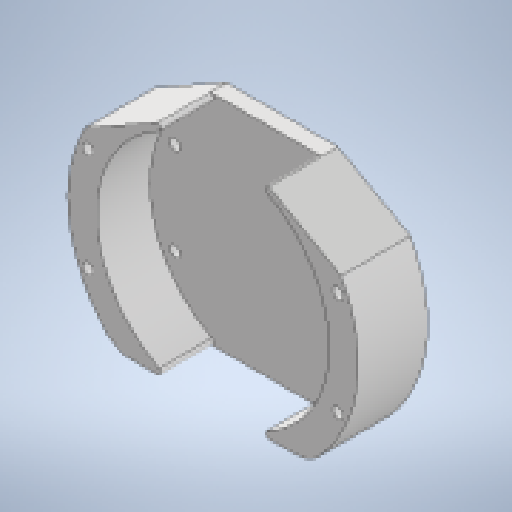
# Autodesk Inventor part: basefixpart_forR6
Saved by Autodesk Inventor 2024.3 (Build 283343010, 343A)
## iProperties
Created: 2025-05-24
Part Number: basefixpart_forR6
Material: 一般
Document SubType Name: Modeling
Designer: kshau
Density: 1 g/cm^3
Appearance: 既定
Mass: 77.9972 g
Surface Area: 271.132 cm^2
Volume: 77.9972 cm^3
Author: kshau
Autodesk Inventor part; units mm, degrees
ref_plane "YZ Plane" through (0, 0, 0) normal (1, 0, 0) x (0, 1, 0)
ref_plane "XZ Plane" through (0, 0, 0) normal (0, 1, 0) x (-1, 0, 0)
ref_plane "XY Plane" through (0, 0, 0) normal (0, 0, 1) x (1, 0, 0)
sketch "スケッチ1" plane through (0, 0, 0) normal (0, 0, 1) x (1, 0, 0)
  circle A0 centre (0, 0) radius 44
  line L0 (0, 0) -> (44, 0)
  line L1 (0, 0) -> (28.9895, 33.1)
  line L2 (28.9895, 33.1) -> (0, 33.1)
  line L3 (0, 0) -> (0, 44)
  line L4 (-28.9895, 33.1) -> (0, 33.1)
  line L5 (28.9895, -33.1) -> (0, -33.1)
  line L6 (-28.9895, -33.1) -> (0, -33.1)
  line L7 (15.4, -33.1) -> (15.4, -41.217)
  line L8 (-15.4, -33.1) -> (-15.4, -41.217)
  line L9 (15.4, 33.1) -> (15.4, 41.217)
  line L10 (-15.4, 33.1) -> (-15.4, 41.217)
  point P0 (-28.9895, 33.1)
  point P1 (-28.9895, -33.1)
  point P2 (28.9895, -33.1)
  point P3 (15.4, 33.1)
  point P4 (-15.4, 33.1)
  point P5 (-15.4, -33.1)
  dimension "d0" = 88
  dimension "d20" = 15.4
  dimension "d21" = 33.1
  constraints: 22 end point, 10 symmetric about line, 4 point on circle, 2 horizontal, 1 centre point, 1 coincident, 1 perpendicular, 1 point on line, 1 vertical
  measures "d0" diameter of A0
  measures "d20" distance between parallel lines of L3 L7
  measures "d21" distance between parallel lines of L0 L2
extrude "押し出し1" add sketch "スケッチ1" along normal blind 5
sketch "スケッチ13" plane through (0, 0, 5) normal (0, 0, 1) x (1, 0, 0)
  circle A0 centre (0, 0) radius 44
  circle A1 centre (0, 0) radius 35.25
  circle A2 centre (0, 0) radius 44 projected
  line L0 (0, 44) -> (0, 0)
  line L1 (7.85, 43.2941) -> (7.85, -43.2941)
  line L2 (-7.85, 43.2941) -> (-7.85, -43.2941)
  point P0 (7.85, -34.3648)
  point P1 (7.85, -43.2941)
  point P2 (7.85, 34.3648)
  point P3 (-7.85, -34.3648)
  point P4 (-7.85, 34.3648)
  dimension "d76" = 88
  dimension "d77" = 70.5
  dimension "d78" = 7.85
  constraints: 6 end point, 3 point on circle, 2 centre point, 2 coincident, 2 symmetric about line, 2 vertical
  measures "d76" diameter of A0
  measures "d77" diameter of A1
  measures "d78" distance between parallel lines of L0 L1
extrude "押し出し9" add sketch "スケッチ13" along normal blind 16 contours A0 L1 A1 | L1 A1 L0 A0 | A0 L2 A1 L1 | L0 A1 L2 A0 | A0 L2 A1
sketch "スケッチ16" plane through (0, 0, 0) normal (0, 0, -1) x (-1, 0, 0)
  line L0 (0, 0) -> (-44, 0)
  circle A0 centre (0, 0) radius 44 projected
  line L1 (0, 0) -> (-40.6507, 16.8381)
  circle A1 centre (0, 0) radius 41
  point P0 (-7.85, -43.2941)
  point P1 (-7.85, 43.2941)
  point P2 (-37.8791, 15.69)
  point P3 (-37.8791, -15.69)
  point P4 (-15.69, -37.8791)
  point P5 (15.69, -37.8791)
  point P6 (37.8791, -15.69)
  point P7 (37.8791, 15.69)
  point P8 (15.69, 37.8791)
  point P9 (-15.69, 37.8791)
  dimension "d92" = 82
  dimension "d91" = 22.5
  dimension "d95" = 360
  constraints: 4 end point, 2 point on circle, 1 coincident, 1 horizontal, 1 point on line, 12 other
  measures "d91" angle of L0 L1
hole "穴5" at (37.8791, 15.69, 0) at (37.8791, -15.69, 0) at (-37.8791, -15.69, 0) at (-37.8791, 15.69, 0) direction (0, 0, 1) diameter 3.3 end through all
sketch "スケッチ19" plane through (0, 0, 0) normal (0, 0, -1) x (-1, 0, 0)
  circle A0 centre (0, 0) radius 31
  line L0 (0, 0) -> (44, 0)
  circle A1 centre (0, 0) radius 44 projected
  line L1 (0, 0) -> (0, 31)
  point P0 (27.6333, 14.05)
  point P1 (27.6333, -14.05)
  point P2 (-27.6333, 14.05)
  point P3 (-27.6333, -14.05)
  dimension "d129" = 62
  dimension "d130" = 14.05
  constraints: 4 end point, 3 symmetric about line, 2 point on circle, 1 centre point, 1 coincident, 1 horizontal, 1 horizontal alignment, 1 vertical, 1 other
  measures "d129" diameter of A0
  measures "d130" distance from line of L0 A0.start
hole "穴6" at (-27.6333, 14.05, 0) at (-27.6333, -14.05, 0) at (27.6333, -14.05, 0) at (27.6333, 14.05, 0) direction (0, 0, 1) diameter 3.3 end through all
sketch "スケッチ21" plane through (0, 0, 0) normal (0, 0, -1) x (-1, 0, 0)
  circle A0 centre (0, 0) radius 17.5
  dimension "d143" = 35
  constraints: 1 centre point, 1 coincident
  measures "d143" diameter of A0
extrude "押し出し15" add sketch "スケッチ21" along normal blind 5
sketch "スケッチ22" plane through (0, 0, -5) normal (0, 0, -1) x (-1, 0, 0)
  circle A0 centre (0, 0) radius 11.15
  dimension "d146" = 22.3
  constraints: 1 centre point, 1 coincident
  measures "d146" diameter of A0
extrude "押し出し16" cut sketch "スケッチ22" against normal blind 6
sketch "スケッチ23" plane through (0, 0, 21) normal (0, 0, 1) x (1, 0, 0)
  circle A0 centre (0, 0) radius 11.15 projected
  line L0 (0, 0) -> (44, 0)
  circle A1 centre (0, 0) radius 44 projected
  line L1 (0, 0) -> (0, 44)
  line L2 (28.9895, 33.1) -> (0, 33.1)
  circle A2 centre (0, 0) radius 44
  line L3 (-28.9895, 33.1) -> (0, 33.1)
  line L4 (28.9895, -33.1) -> (0, -33.1)
  line L5 (-28.9895, -33.1) -> (0, -33.1)
  dimension "d151" = 33.1
  constraints: 12 end point, 4 symmetric about line, 3 point on circle, 1 centre point, 1 coincident, 1 concentric, 1 horizontal, 1 perpendicular, 1 point on line, 1 vertical
  measures "d151" distance between parallel lines of L0 L2
extrude "押し出し17" cut sketch "スケッチ23" against normal blind 25 contours L3 A1 L1 | L1 A1 L2 | A1 L5 L4
sketch "スケッチ24" plane through (0, 0, 0) normal (0, 0, -1) x (-1, 0, 0)
  circle A0 centre (0, 0) radius 11.15 projected
  circle A1 centre (0, 0) radius 59
  arc A2 (28.9895, -33.1) -> (28.9895, 33.1) centre (0, 0) ccw projected
  line L0 (12.1224, 33.1) -> (28.9895, 33.1) projected
  line L1 (28.9895, 33.1) -> (48.8405, 33.1)
  line L2 (-28.9895, 33.1) -> (-48.8405, 33.1)
  arc A3 (-28.9895, 33.1) -> (-28.9895, -33.1) centre (0, 0) ccw projected
  line L3 (-28.9895, -33.1) -> (-48.8405, -33.1)
  line L4 (28.9895, -33.1) -> (48.8405, -33.1)
  dimension "d154" = 15
  constraints: 8 end point, 3 point on circle, 2 point on line, 1 centre point, 1 coincident, 1 collinear, 1 horizontal, 1 parallel
  measures "d154" radial gap between concentric circles of A2 A1
extrude "押し出し18" [suppressed]
sketch "スケッチ25" plane through (0, 0, 5) normal (0, 0, 1) x (1, 0, 0)
  circle A0 centre (0, 0) radius 11.15 projected
  arc A1 (-48.8405, 33.1) -> (-48.8405, -33.1) centre (0, 0) ccw projected
  circle A2 centre (0, 0) radius 59
  circle A3 centre (0, 0) radius 54
  line L0 (-48.8405, 33.1) -> (48.8405, 33.1) projected
  line L1 (-48.8405, 33.1) -> (48.8405, 33.1)
  line L2 (48.8405, -33.1) -> (-48.8405, -33.1) projected
  line L3 (48.8405, -33.1) -> (-48.8405, -33.1)
  point P0 (-42.666, -33.1)
  point P1 (-42.666, 33.1)
  point P2 (42.666, -33.1)
  point P3 (42.666, 33.1)
  dimension "d157" = 5
  constraints: 4 end point, 2 centre point, 2 coincident, 1 collinear, 1 horizontal, 1 point on circle
  measures "d157" radial gap between concentric circles of A1 A3
extrude "押し出し19" [suppressed]
fillet "フィレット19" radius 10 1 edges at (17.5, 0, 0)
fillet "フィレット20" radius 1 2 edges at (17.5, 0, -5) (11.15, 0, -5)
fillet "フィレット21" radius 1 4 edges at (12.1224, 33.1, 13) (-12.1224, 33.1, 13) (12.1224, -33.1, 13) (-12.1224, -33.1, 13)
fillet "フィレット22" radius 10 4 edges at (-28.9895, 33.1, 10.5) (28.9895, 33.1, 10.5) (28.9895, -33.1, 10.5) (-28.9895, -33.1, 10.5)
sketch "スケッチ26" plane through (0, 0, 0) normal (0, 0, -1) x (-1, 0, 0)
  arc A0 (-32.2853, 29.8941) -> (-32.2853, -29.8941) centre (0, 0) ccw projected
  line L0 (-38.832, 20.69) -> (-16.832, 33.1)
  line L1 (24.9477, 33.1) -> (-24.9477, 33.1) projected
  line L2 (-38.832, 20.69) -> (38.832, 20.69)
  arc A1 (32.2853, -29.8941) -> (32.2853, 29.8941) centre (0, 0) ccw projected
  circle A2 centre (-37.8791, 15.69) radius 1.65 projected
  line L3 (-38.832, 20.69) -> (-16.832, 20.69)
  line L4 (-16.832, 20.69) -> (-16.832, 33.1)
  line L5 (-16.832, 33.1) -> (-38.832, 33.1)
  line L6 (-38.832, 33.1) -> (-38.832, 20.69)
  line L7 (0, 0) -> (0, 33.1)
  line L8 (-16.842, 33.1) -> (16.842, 33.1) projected
  line L9 (38.832, 20.69) -> (16.832, 33.1)
  line L10 (16.832, 20.69) -> (16.832, 33.1)
  line L11 (16.832, 33.1) -> (38.832, 33.1)
  line L12 (38.832, 33.1) -> (38.832, 20.69)
  point P0 (-24.9477, 33.1)
  dimension "d164" = 5
  dimension "d165" = 22
  constraints: 22 end point, 3 symmetric about line, 2 horizontal, 2 parallel, 2 point on circle, 1 midpoint, 1 perpendicular, 1 point on line
  measures "d164" distance from line of A2.centre L2
  measures "d165" distance between parallel lines of L6 L4
extrude "押し出し20" cut sketch "スケッチ26" against normal blind 25 contours L6 L5 L1 L0 | L1 L11 L12 L9
